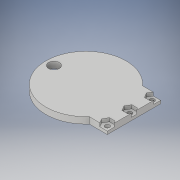
# Autodesk Inventor part: feeder_base
Saved by Autodesk Inventor 2019 (Build 230136000, 136)
## iProperties
Created: 2018-11-15
Part Number: feeder_base
Material: Generic
Document SubType Name: Modeling
Designer: chill
Density: 1 g/cm^3
Appearance: Default
Author: chill
Autodesk Inventor part; units mm, degrees
ref_plane "YZ Plane" through (0, 0, 0) normal (1, 0, 0) x (0, 1, 0)
ref_plane "XZ Plane" through (0, 0, 0) normal (0, 1, 0) x (-1, 0, 0)
ref_plane "XY Plane" through (0, 0, 0) normal (0, 0, 1) x (1, 0, 0)
sketch "Sketch1" plane through (0, 0, 0) normal (0, 1, 0) x (-1, 0, 0)
  arc A0 (-27.9508, -25) -> (-27.9508, 25) centre (0, 0) ccw
  circle A1 centre (30, 0) radius 5
  line L0 (-27.9508, 25) -> (-45, 25)
  line L1 (-27.9508, -25) -> (-45, -25)
  line L2 (-45, 25) -> (-45, -25)
  line L3 (30, 0) -> (0, 0)
  dimension "d0" = 75
  dimension "d1" = 10
  dimension "d2" = 30
  dimension "d3" = 25
  dimension "d4" = 25
  dimension "d6" = 45
  constraints: 8 end point, 3 horizontal, 2 centre point, 2 point on circle, 1 coincident, 1 vertical
  measures "d0" diameter of A0
  measures "d1" diameter of A1
  measures "d2" distance of L3.start point (0, 0)
  measures "d3" distance from line of L0 point (0, 0)
  measures "d4" distance from line of L1 point (0, 0)
  measures "d6" distance from line of L2 point (0, 0)
extrude "Extrusion1" add sketch "Sketch1" along normal blind 6
sketch "Sketch2" plane through (0, 6, 0) normal (0, 1, 0) x (1, 0, 0)
  circle A0 centre (-30, 0) radius 5 projected
  line L0 (27.9508, -25) -> (45, -25) projected
  line L1 (45, -25) -> (45, 25) projected
  line L2 (45, 25) -> (27.9508, 25) projected
  arc A1 (27.9508, 25) -> (27.9508, -25) centre (0, 0) ccw projected
  circle A2 centre (41, -21) radius 2.125
  circle A3 centre (41, 21) radius 2.125
  circle A4 centre (41, 0) radius 2.125
  dimension "d15" = 4.25
  dimension "d16" = 4.25
  dimension "d17" = 4.25
  dimension "d18" = 4
  dimension "d19" = 4
  dimension "d20" = 4
  dimension "d21" = 4
  dimension "d22" = 4
  dimension "d23" = 41
  constraints: 3 centre point
  measures "d15" diameter of A2
  measures "d16" diameter of A3
  measures "d17" diameter of A4
  measures "d18" distance from line of L0 A2.centre
  measures "d19" distance from line of A2.centre L1
  measures "d20" distance from line of L1 A4.centre
  measures "d21" distance from line of L2 A3.centre
  measures "d22" distance from line of L1 A3.centre
  measures "d23" distance of point (0, 0) A4.centre
extrude "Extrusion2" cut sketch "Sketch2" against normal through all contours A2 | A3 | A4
sketch "Sketch4" plane through (0, 6, 0) normal (0, 1, 0) x (1, 0, 0)
  circle A0 centre (41, 21) radius 2.125 projected
  circle A1 centre (41, 0) radius 2.125 projected
  circle A2 centre (41, -21) radius 2.125 projected
  line L0 (43.6702, 25.625) -> (46.3405, 21)
  line L1 (46.3405, 21) -> (43.6702, 16.375)
  line L2 (43.6702, 16.375) -> (38.3298, 16.375)
  line L3 (38.3298, 16.375) -> (35.6595, 21)
  line L4 (35.6595, 21) -> (38.3298, 25.625)
  line L5 (38.3298, 25.625) -> (43.6702, 25.625)
  line L6 (43.6702, 4.625) -> (46.3405, 0)
  line L7 (46.3405, 0) -> (43.6702, -4.625)
  line L8 (43.6702, -4.625) -> (38.3298, -4.625)
  line L9 (38.3298, -4.625) -> (35.6595, 0)
  line L10 (35.6595, 0) -> (38.3298, 4.625)
  line L11 (38.3298, 4.625) -> (43.6702, 4.625)
  line L12 (43.6702, -16.375) -> (46.3405, -21)
  line L13 (46.3405, -21) -> (43.6702, -25.625)
  line L14 (43.6702, -25.625) -> (38.3298, -25.625)
  line L15 (38.3298, -25.625) -> (35.6595, -21)
  line L16 (35.6595, -21) -> (38.3298, -16.375)
  line L17 (38.3298, -16.375) -> (43.6702, -16.375)
  point P0 (0, 0)
  point P1 (41, 25.625)
  point P2 (41, 4.625)
  point P3 (41, -16.375)
  dimension "d35" = 9.25
  dimension "d36" = 9.25
  dimension "d37" = 9.25
  dimension "d38" = 21
  dimension "d39" = 42
  dimension "d40" = 4.625
  dimension "d41" = 4.625
  dimension "d42" = 5.875
  dimension "d43" = 16.375
  constraints: 36 end point, 3 midpoint, 2 parallel, 1 horizontal, 39 other
  measures "d35" distance between parallel lines of L1 L4
  measures "d36" distance between parallel lines of L7 L10
  measures "d37" distance between parallel lines of L12 L15
  measures "d38" distance between parallel lines of L5 L11
  measures "d39" distance between parallel lines of L5 L17
  measures "d40" distance from line of A0.centre L0
  measures "d41" distance from line of A0.centre L1
  measures "d42" distance from line of A0.centre L6
  measures "d43" distance from line of A0.centre L12
extrude "Extrusion4" cut sketch "Sketch4" against normal blind 3.25
sketch "Sketch5" plane through (0, 6, 0) normal (0, 1, 0) x (1, 0, 0)
  line L0 (44.0311, 25) -> (45, 23.3218) projected
  line L1 (45, 23.3218) -> (45, 25) projected
  line L2 (45, 25) -> (44.0311, 25) projected
  line L3 (45, -23.3218) -> (44.0311, -25) projected
  line L4 (45, -23.3218) -> (44.0311, -25) projected
  line L5 (44.0311, -25) -> (45, -25) projected
  line L6 (45, -25) -> (45, -23.3218) projected
  point P0 (0, 0)
extrude "Extrusion5" cut sketch "Sketch5" against normal blind 3.25
body "Solid1"
